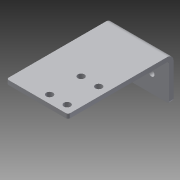
# Autodesk Inventor part: Pneumatic Piston Back Flange (Right Custom)
Saved by Autodesk Inventor 2014 (Build 180170000, 170)
## iProperties
Created: 2014-01-13
Part Number: Pneumatic Piston Back Flange (Right Custom)
Material: Generic
Document SubType Name: Sheet Metal
Designer: motoennies
Density: 1 g/cm^3
Sheet Metal Rule: Default
Appearance: Default
Author: motoennies
Autodesk Inventor part; units mm, degrees
ref_plane "YZ Plane" through (0, 0, 0) normal (1, 0, 0) x (0, 1, 0)
ref_plane "XZ Plane" through (0, 0, 0) normal (0, 1, 0) x (-1, 0, 0)
ref_plane "XY Plane" through (0, 0, 0) normal (0, 0, 1) x (1, 0, 0)
sketch "Sketch1" plane through (0, 0, 0) normal (0, 0, 1) x (1, 0, 0)
  line L0 (0, 0) -> (44.45, 0)
  line L1 (44.45, 0) -> (44.45, 25.4)
  line L2 (44.45, 25.4) -> (0, 25.4)
  line L3 (0, 25.4) -> (0, 0)
  circle A0 centre (6.35, 12.7) radius 2.0701
  line L4 (0, 12.7) -> (44.45, 12.7) construction
  circle A1 centre (31.75, 12.7) radius 2.0701
  dimension "d0" = 44.45
  dimension "d1" = 25.4
  dimension "d2" = 4.1402
  dimension "d6" = 25.4
  dimension "d34" = 6.35
  measures "d0" distance of L2.end L1.end
  measures "d1" distance of L1.end L0.end
  measures "d2" diameter of A0
  measures "d6" distance of A0.centre A1.centre
  measures "d34" distance from line of L3 A0.centre
extrude "Plate1" add sketch "Sketch1" along normal blind 3.175
sketch "Sketch2" plane through (0, 26.67, 4.445) normal (0, 1, 0) x (-1, 0, 0)
  line L0 (-44.45, 0) -> (0, 0)
  line L1 (0, 0) -> (0, 71.755)
  line L2 (0, 71.755) -> (-44.45, 71.755)
  line L3 (-44.45, 71.755) -> (-44.45, 0)
  constraints: 6 end point, 1 horizontal, 1 perpendicular, 1 vertical
edge flange "Flange1" height 76.2 angle 90 thickness 3.175 bend radius 1.27 thickness toward (0, 1, 0) relief straight relief width 3.175 relief depth 1.5875 edges at (22.225, 25.4, 3.175) wall of the first edge with corners at (44.45, 26.67, 4.445) (0, 26.67, 4.445) (0, 26.67, 76.2) (44.45, 26.67, 76.2)
bend "Bend1"
corner "Corner1"
fillet "Fillet1" radius 1.5875 4 edges at (44.45, 0, 1.5875) (0, 0, 1.5875) (0, 28.2575, 76.2) (44.45, 28.2575, 76.2)
sketch "Sketch3" plane through (0, 26.67, 4.445) normal (0, -1, 0) x (1, 0, 0)
  line L0 (22.225, 71.755) -> (41.275, 71.755) construction
  line L1 (41.275, 71.755) -> (41.275, 37.465) construction
  line L2 (41.275, 37.465) -> (22.225, 37.465) construction
  line L3 (22.225, 37.465) -> (22.225, 71.755) construction
  circle A0 centre (38.1, 66.0019) radius 2.413
  line L4 (31.75, 71.755) -> (31.75, 37.465) construction
  line L5 (22.225, 54.61) -> (41.275, 54.61) construction
  circle A1 centre (25.4, 66.0019) radius 2.413
  circle A2 centre (38.1, 43.2181) radius 2.413
  circle A3 centre (25.4, 43.2181) radius 2.413
  line L6 (42.8625, 71.755) -> (1.5875, 71.755) projected
  line L7 (0, 70.1675) -> (0, 0) projected
  point P0 (0, -4.445)
  dimension "d23" = 34.29
  dimension "d24" = 19.05
  dimension "d27" = 4.826
  dimension "d28" = 3.175
  dimension "d29" = 5.7531
  dimension "d35" = 22.225
  constraints: 12 end point, 4 centre point, 4 midpoint, 3 symmetric about line, 2 parallel, 1 collinear, 1 horizontal, 1 perpendicular, 3 other
  measures "d23" distance of L2.end L0.start
  measures "d24" distance of L0.start L0.end
  measures "d27" diameter of A0
  measures "d28" distance from line of L1 A0.centre
  measures "d29" distance from line of A0.centre L0
  measures "d35" distance between parallel lines of L7 L3
extrude "Extrusion1" cut sketch "Sketch3" against normal blind 25.4
equation "\"d12\" = BendReliefWidth"
equation "\"d13\" = BendReliefDepth"
equation "\"d14\" = MinimumRemnant"
equation "\"d15\" = BendRadius"
equation "\"d19\" = CornerReliefSize"
equation "\"d20\" = GapSize"
equation "\"d21\" = JacobiRadiusSize"
equation "\"BendRadius\" = Thickness"
equation "\"BendReliefWidth\" = Thickness"
equation "\"BendReliefDepth\" = 0.5 * Thickness"
equation "\"CornerReliefSize\" = 4 * Thickness"
equation "\"MinimumRemnant\" = 2 * Thickness"
equation "\"TransitionRadius\" = BendRadius"
equation "\"JacobiRadiusSize\" = BendRadius"
equation "\"GapSize\" = Thickness"
equation "\"d11\" = BendRadius"
equation "\"Thickness\" = 3.175"
body "Solid1"
